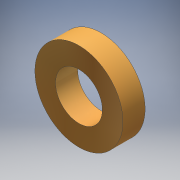
# Autodesk Inventor part: MotorSiliconeMoldSpacer
Saved by Autodesk Inventor 2016 (Build 200138000, 138)
## iProperties
Created: 2015-12-05
Part Number: MotorSiliconeMoldSpacer
Material: Plywood, Sheathing
Document SubType Name: Modeling
Designer: DonMo
Density: 0.552 g/cm^3
Appearance: Plywood - New
Author: DonMo
Autodesk Inventor part; units mm, degrees
ref_plane "YZ Plane" through (0, 0, 0) normal (1, 0, 0) x (0, 1, 0)
ref_plane "XZ Plane" through (0, 0, 0) normal (0, 1, 0) x (-1, 0, 0)
ref_plane "XY Plane" through (0, 0, 0) normal (0, 0, 1) x (1, 0, 0)
sketch "Sketch1" plane through (0, 0, 0) normal (0, 1, 0) x (-1, 0, 0)
  circle A0 centre (0, 0) radius 3.175
  circle A1 centre (0, 0) radius 5.9688
  dimension "d0" = 6.35
  dimension "d1" = 11.9375
  constraints: 2 centre point, 2 coincident
  measures "d0" diameter of A0
  measures "d1" diameter of A1
extrude "Extrusion1" add sketch "Sketch1" along normal blind 3
equation "\"d0\" = DowlDiameter"
equation "\"DowlDiameter\" = 6.35"
body "Solid1"
